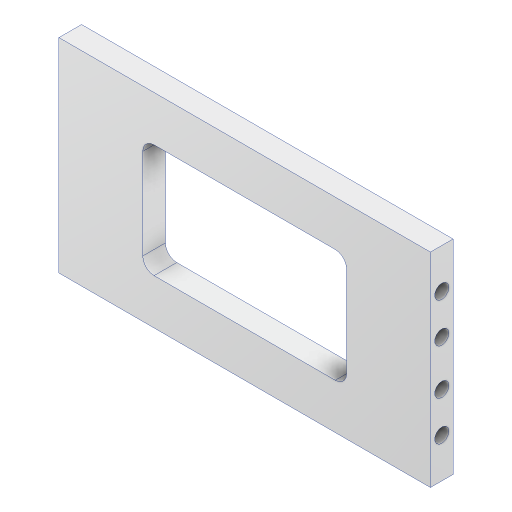
# Autodesk Inventor part: 지지프레임1
Saved by Autodesk Inventor 2023.2 (Build 272271000, 271)
## iProperties
Created: 2022-12-28
Part Number: 지지프레임1
Material: 알루미늄 6061
Document SubType Name: Modeling
Designer: BAEK
Density: 2.7 g/cm^3
Appearance: 알루미늄 - 평지
Mass: 13.9161 g
Surface Area: 40.5012 cm^2
Volume: 5.15412 cm^3
Author: BAEK
Autodesk Inventor part; units mm, degrees
ref_plane "YZ Plane" through (0, 0, 0) normal (1, 0, 0) x (0, 1, 0)
ref_plane "XZ Plane" through (0, 0, 0) normal (0, 1, 0) x (-1, 0, 0)
ref_plane "XY Plane" through (0, 0, 0) normal (0, 0, 1) x (1, 0, 0)
sketch "스케치1" plane through (0, 0, 0) normal (0, 0, 1) x (1, 0, 0)
  line L0 (-32.8, 18) -> (32.8, 18)
  line L1 (32.8, 18) -> (32.8, -18)
  line L2 (32.8, -18) -> (-32.8, -18)
  line L3 (-32.8, -18) -> (-32.8, 18)
  line L4 (-32.8, 18) -> (32.8, -18) construction
  line L5 (32.8, 18) -> (-32.8, -18) construction
  point P0 (0, 0)
  dimension "d0" = 65.6
  dimension "d1" = 36
  constraints: 12 end point, 2 midpoint, 2 parallel, 1 horizontal, 1 perpendicular
  measures "d0" distance of L1.end L2.end
  measures "d1" distance of L0.end L1.end
extrude "돌출1" add sketch "스케치1" along normal blind 4
sketch "스케치2" plane through (32.8, -18, 0) normal (1, 0, 0) x (0, 0, -1)
  line L0 (0, 0) -> (0, 36) projected
  line L1 (0, 36) -> (-4, 36) projected
  line L2 (-4, 0) -> (-4, 36) projected
  line L3 (0, 0) -> (-4, 0) projected
  line L4 (0, 0) -> (-4, 0) projected
  line L5 (-2, 0) -> (-2, 36) construction
  line L6 (0, 36) -> (-4, 36) projected
  circle A0 centre (-2, 7) radius 1.25
  circle A1 centre (-2, 14) radius 1.25
  circle A2 centre (-2, 22) radius 1.25
  circle A3 centre (-2, 29) radius 1.25
  point P0 (0, 18)
  dimension "d4" = 2.5
  dimension "d5" = 2.5
  dimension "d7" = 2.5
  dimension "d8" = 7
  dimension "d9" = 7
  dimension "d11" = 2.5
  dimension "d12" = 7
  dimension "d13" = 7
  constraints: 4 centre point, 4 point on line, 2 end point, 2 midpoint
  measures "d4" diameter of A0
  measures "d5" diameter of A1
  measures "d7" diameter of A2
  measures "d8" distance from line of L3 A0.centre
  measures "d9" distance of A0.centre A1.centre
  measures "d11" diameter of A3
  measures "d12" distance from line of L1 A3.centre
  measures "d13" distance of A2.centre A3.centre
extrude "돌출2" cut sketch "스케치2" against normal blind 6 contours A0 | A1 | A2 | A3
mirror "미러1" about plane through (0, 0, 0) normal (1, 0, 0) of "돌출2"
sketch "스케치3" plane through (0, 0, 4) normal (0, 0, 1) x (1, 0, 0)
  line L0 (18, -10) -> (-18, -10)
  line L1 (-18, -10) -> (-18, 10)
  line L2 (-18, 10) -> (18, 10)
  line L3 (18, 10) -> (18, -10)
  line L4 (18, -10) -> (-18, 10) construction
  line L5 (-18, -10) -> (18, 10) construction
  point P0 (0, 0)
  dimension "d16" = 36
  dimension "d17" = 20
  constraints: 12 end point, 2 midpoint, 2 parallel, 1 horizontal, 1 perpendicular
  measures "d16" distance of L1.end L2.end
  measures "d17" distance of L0.end L1.end
extrude "돌출3" cut sketch "스케치3" against normal blind 6
fillet "모깎기1" radius 2 4 edges at (18, -10, 2) (18, 10, 2) (-18, 10, 2) (-18, -10, 2)
